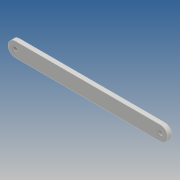
# Autodesk Inventor part: Front guard
Saved by Autodesk Inventor 2017 (Build 210142000, 142)
## iProperties
Created: 2017-07-08
Part Number: Front guard
Material: Generic
Document SubType Name: Modeling
Designer: yella
Density: 1 g/cm^3
Appearance: Default
Author: yella
Autodesk Inventor part; units mm, degrees
ref_plane "YZ Plane" through (0, 0, 0) normal (1, 0, 0) x (0, 1, 0)
ref_plane "XZ Plane" through (0, 0, 0) normal (0, 1, 0) x (-1, 0, 0)
ref_plane "XY Plane" through (0, 0, 0) normal (0, 0, 1) x (1, 0, 0)
sketch "Sketch1" plane through (0, 0, 0) normal (0, 1, 0) x (-1, 0, 0)
  circle A0 centre (50.4794, -84.4325) radius 1.6
  circle A1 centre (-50.4794, -84.4325) radius 1.6
  arc A2 (50.4794, -89.4325) -> (50.4794, -79.4325) centre (50.4794, -84.4325) ccw
  arc A3 (-50.4794, -79.4325) -> (-50.4794, -89.4325) centre (-50.4794, -84.4325) ccw
  line L0 (50.4794, -79.4325) -> (-50.4794, -79.4325)
  line L1 (-50.4794, -89.4325) -> (50.4794, -89.4325)
  point P0 (0, 0)
  dimension "d0" = 3.2
  dimension "d1" = 3.2
  dimension "d2" = 5
  dimension "d3" = 5
  constraints: 4 centre point, 4 coincident, 4 end point, 4 point on circle, 1 horizontal, 1 parallel
  measures "d0" diameter of A0
  measures "d1" diameter of A1
  measures "d2" radius of A2
  measures "d3" radius of A3
extrude "Extrusion1" add sketch "Sketch1" along normal blind 3
body "Solid1"
